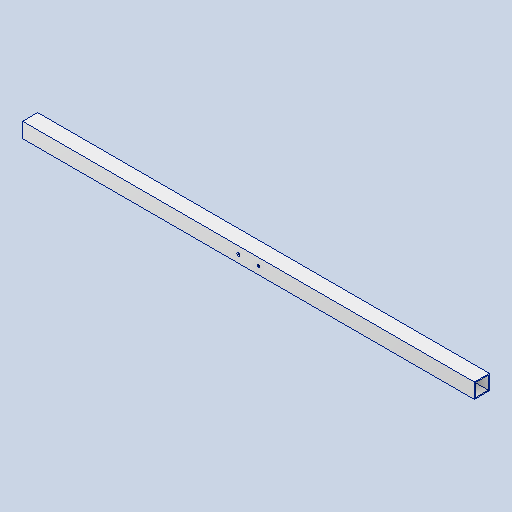
# Autodesk Inventor part: hand-grab-v2-ASP-arm-support
Saved by Autodesk Inventor 2025.1 (Build 291241000, 241)
## iProperties
Created: 2024-10-21
Part Number: hand-grab-v2-ASP-arm-support
Material: アルミニウム 6061
Document SubType Name: Modeling
Designer: haruy
Density: 2.7 g/cm^3
Appearance: アルミニウム - フラット
Author: haruy
Autodesk Inventor part; units mm, degrees
ref_plane "YZ Plane" through (0, 0, 0) normal (1, 0, 0) x (0, 1, 0)
ref_plane "XZ Plane" through (0, 0, 0) normal (0, 1, 0) x (-1, 0, 0)
ref_plane "XY Plane" through (0, 0, 0) normal (0, 0, 1) x (1, 0, 0)
sketch "スケッチ1" plane through (0, 0, 0) normal (1, 0, 0) x (0, 1, 0)
  line L0 (0, 0) -> (15, 0)
  line L1 (15, 0) -> (15, -15)
  line L2 (15, -15) -> (0, -15)
  line L3 (0, -15) -> (0, 0)
  line L4 (14, -1) -> (1, -1)
  line L5 (1, -1) -> (1, -14)
  line L6 (1, -14) -> (14, -14)
  line L7 (14, -14) -> (14, -1)
  dimension "d0" = 15
  dimension "d1" = 15
  dimension "d2" = 1
  constraints: 16 end point, 4 parallel, 2 perpendicular, 1 horizontal, 3 other
  measures "d0" distance of L1.end L2.end
  measures "d1" distance of L0.end L1.end
  measures "d2" distance between parallel lines of L0 L4
extrude "押し出し1" add sketch "スケッチ1" along normal blind 450
sketch "スケッチ2" plane through (0, 0, 0) normal (0, 0, 1) x (1, 0, 0)
  line L0 (0, 15) -> (450, 15) projected
  line L1 (225, 15) -> (225, 0)
  line L2 (0, 15) -> (0, 0) projected
  point P0 (215, 7.5)
  point P1 (235, 7.5)
  dimension "d5" = 225
  dimension "d6" = 10
  dimension "d7" = 10
  dimension "d8" = 7.5
  dimension "d9" = 7.5
  constraints: 2 end point, 1 midpoint, 1 vertical
  measures "d5" distance between parallel lines of L2 L1
  measures "d6" distance from line of point (215, 7.5) L1
  measures "d7" distance from line of point (235, 7.5) L1
  measures "d8" distance from line of point (215, 7.5) L0
  measures "d9" distance from line of point (235, 7.5) L0
hole "穴1" at (215, 7.5, 0) at (235, 7.5, 0) direction (0, 0, -1) diameter 3 end through all
